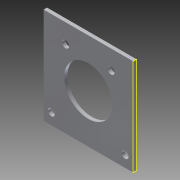
# Autodesk Inventor part: upper face mount
Saved by Autodesk Inventor 2013 (Build 170138000, 138)
## iProperties
Created: 2013-01-24
Part Number: upper face mount
Material: Aluminum 6061
Document SubType Name: Sheet Metal
Designer: Arpan
Density: 2.71 g/cm^3
Sheet Metal Rule: Default
Mass: 25.8694 g
Surface Area: 70.3767 cm^2
Volume: 9.54591 cm^3
Author: Arpan
Autodesk Inventor part; units mm, degrees
ref_plane "YZ Plane" through (0, 0, 0) normal (1, 0, 0) x (0, 1, 0)
ref_plane "XZ Plane" through (0, 0, 0) normal (0, 1, 0) x (-1, 0, 0)
ref_plane "XY Plane" through (0, 0, 0) normal (0, 0, 1) x (1, 0, 0)
sketch "Sketch1" plane through (0, 0, 0) normal (0, 0, 1) x (1, 0, 0)
  line L0 (0, 0) -> (-56.9976, 0)
  line L1 (-56.9976, 88.9) -> (0, 88.9)
  line L2 (0, 88.9) -> (-7.493, 88.9)
  line L3 (-7.493, 88.9) -> (-7.493, 82.55)
  line L4 (-56.9976, 88.9) -> (-49.5046, 88.9)
  line L5 (-49.5046, 88.9) -> (-49.5046, 82.55)
  line L6 (-56.9976, 88.9) -> (-69.6976, 88.9)
  line L7 (-69.6976, 88.9) -> (-69.6976, 0)
  line L8 (-69.6976, 0) -> (-56.9976, 0)
  line L9 (0, 88.9) -> (8.89, 88.9)
  line L10 (8.89, 0) -> (0, 0)
  line L11 (0, 88.9) -> (12.7, 88.9)
  line L12 (12.7, 88.9) -> (12.7, 0)
  line L13 (12.7, 0) -> (0, 0)
  dimension "d1" = 56.9976
  dimension "d2" = 88.9
  dimension "d3" = 7.493
  dimension "d4" = 6.35
  dimension "d5" = 7.493
  dimension "d19" = 6.35
  dimension "d48" = 12.7
  dimension "d57" = 12.7
  constraints: 28 end point, 4 perpendicular, 3 parallel, 3 point on line, 2 collinear, 1 horizontal
  measures "d1" distance of L0.start L0.end
  measures "d2" distance of L0.end L1.start
  measures "d3" distance of L1.end L2.end
  measures "d4" distance of L2.end L3.end
  measures "d5" distance of L1.start L4.end
  measures "d19" distance of L4.end L5.end
  measures "d48" distance of L1.start L6.end
  measures "d57" distance of L1.end L11.end
extrude "Plate5" add sketch "Sketch1" along normal blind 3.175
sketch "Sketch7" plane through (12.7, 0, 0) normal (1, 0, 0) x (0, 0, -1)
  line L0 (-3.175, 88.9) -> (-3.175, 0) projected
  line L1 (0, 0) -> (-3.175, 0) projected
  line L2 (0, 0) -> (0, 88.9) projected
  line L3 (0, 88.9) -> (-3.175, 88.9) projected
sketch "Sketch11" plane through (0, 0, 3.175) normal (0, 0, 1) x (1, 0, 0)
  circle A0 centre (-7.4976, 71.4155) radius 3.3
  circle A1 centre (-49.4976, 71.4155) radius 3.3
  circle A2 centre (5.484, 10.4813) radius 3.2
  line L0 (-11.9976, 581.6155) -> (-11.9976, -78.7845)
  circle A3 centre (5.484, 10.4813) radius 3.2
  line L1 (-53.516, -9.5187) -> (-68.516, -9.5187)
  line L2 (-68.516, 30.4813) -> (-68.516, -9.5187)
  line L3 (-68.516, 30.4813) -> (-53.516, 30.4813)
  line L4 (-53.516, 30.4813) -> (-53.516, -9.5187)
  circle A4 centre (-62.516, 10.4813) radius 3.2
  circle A5 centre (-62.516, 10.4813) radius 3.2
  point P0 (0, 0)
  point P1 (-28.516, 7.2815)
extrude "Cut5" cut sketch "Sketch11" against normal blind 3.175 contours A0 | A1 | A2 | A4
sketch "Sketch12" plane through (0, 0, 3.175) normal (0, 0, 1) x (1, 0, 0)
  line L0 (-69.6976, 88.9) -> (12.7, 88.9) projected
  line L1 (-69.6976, 0) -> (-69.6976, 88.9) projected
  line L2 (-28.4988, 88.9) -> (-28.4988, 44.45)
  circle A0 centre (-28.4988, 44.45) radius 22.225
  point P0 (0, 0)
  dimension "d71" = 44.45
  constraints: 2 end point, 1 centre point, 1 coincident, 1 midpoint, 1 parallel
  measures "d71" diameter of A0
extrude "Cut6" cut sketch "Sketch12" against normal blind 3.175
equation "\"d69\" = Thickness"
equation "\"d72\" = Thickness"
equation "\"BendRadius\" = Thickness"
equation "\"BendReliefWidth\" = Thickness"
equation "\"BendReliefDepth\" = 0.5 * Thickness"
equation "\"CornerReliefSize\" = 4 * Thickness"
equation "\"MinimumRemnant\" = 2 * Thickness"
equation "\"TransitionRadius\" = BendRadius"
equation "\"JacobiRadiusSize\" = BendRadius"
equation "\"GapSize\" = Thickness"
equation "\"d8\" = BendRadius"
equation "\"d56\" = BendRadius"
equation "\"Thickness\" = 3.175"
body "Solid2"
